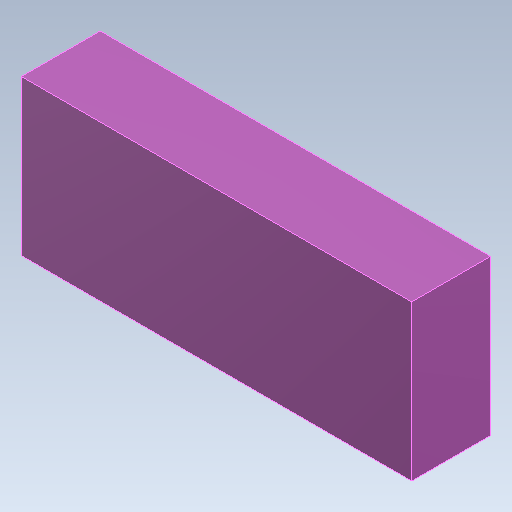
# Autodesk Inventor part: R1206
Saved by Autodesk Inventor 2021 (Build 250183000, 183)
## iProperties
Created: 2020-11-18
Part Number: R1206
Material: Generic
Document SubType Name: Modeling
Designer: Admin
Density: 1 g/cm^3
Appearance: R1206, R1206
Author: Admin
Autodesk Inventor part; units mm, degrees
ref_plane "YZ Plane" through (0, 0, 0) normal (1, 0, 0) x (0, 1, 0)
ref_plane "XZ Plane" through (0, 0, 0) normal (0, 1, 0) x (-1, 0, 0)
ref_plane "XY Plane" through (0, 0, 0) normal (0, 0, 1) x (1, 0, 0)
sketch "R1206, R1206_18" plane through (0, 0, 0) normal (0, 0, 1) x (1, 0, 0)
  line L0 (-2.473, 0.983) -> (2.473, 0.983)
  line L1 (2.473, 0.983) -> (2.473, -0.983)
  line L2 (2.473, -0.983) -> (-2.473, -0.983)
  line L3 (-2.473, -0.983) -> (-2.473, 0.983)
  constraints: 8 end point
extrude "Extrusion1" add sketch "R1206, R1206_18" along normal blind 1
body "Solid1"
